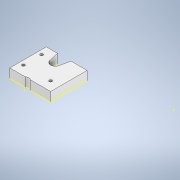
# Autodesk Inventor part: delrin for sides
Saved by Autodesk Inventor 2020.1 (Build 241239000, 239)
## iProperties
Created: 2019-11-10
Part Number: delrin for sides
Material: UHMW, White
Document SubType Name: Modeling
Designer: amirs
Density: 0.94 g/cm^3
Appearance: Smooth - White
Mass: 4.35466 g
Surface Area: 23.8857 cm^2
Volume: 4.63262 cm^3
Author: amirs
Autodesk Inventor part; units mm, degrees
ref_plane "YZ Plane" through (0, 0, 0) normal (1, 0, 0) x (0, 1, 0)
ref_plane "XZ Plane" through (0, 0, 0) normal (0, 1, 0) x (-1, 0, 0)
ref_plane "XY Plane" through (0, 0, 0) normal (0, 0, 1) x (1, 0, 0)
sketch "Sketch1" plane through (0, 0, 0) normal (0, 1, 0) x (-1, 0, 0)
  circle A0 centre (73.1106, 19.0179) radius 0.9652
  circle A1 centre (73.1106, 31.7179) radius 0.9652
  circle A2 centre (54.1114, 31.7179) radius 0.9652
  line L0 (58.8995, 12.6679) -> (60.5161, 19.7267)
  arc A3 (66.7058, 19.7267) -> (60.5161, 19.7267) centre (63.611, 19.0179) ccw
  line L1 (66.7058, 19.7267) -> (68.3224, 12.6679)
  arc A4 (61.706, 38.0679) -> (65.516, 38.0679) centre (63.611, 40.6079) ccw
  line L2 (79.486, 38.0679) -> (79.486, 12.6679) construction
  line L3 (47.736, 12.6679) -> (47.736, 38.0679)
  line L4 (47.736, 38.0679) -> (61.706, 38.0679)
  line L5 (65.516, 38.0679) -> (79.486, 38.0679) construction
  line L6 (79.486, 12.6679) -> (68.3224, 12.6679) construction
  line L7 (58.8995, 12.6679) -> (47.736, 12.6679)
  line L8 (76.184, 38.0679) -> (76.184, 12.6679)
  line L9 (65.516, 38.0679) -> (76.184, 38.0679)
  line L10 (68.3224, 12.6679) -> (76.184, 12.6679)
  point P0 (0, 0)
  dimension "d9" = 1.9304
  dimension "d10" = 25.4
  dimension "d11" = 31.75
  dimension "d14" = 18.9992
  dimension "d15" = 6.3754
  dimension "d16" = 15.875
  dimension "d17" = 15.875
  dimension "d18" = 28.448
  constraints: 22 end point, 5 centre point, 5 parallel, 4 perpendicular, 4 point on circle, 2 equal radius, 2 horizontal, 2 point on line, 1 collinear, 1 vertical alignment
  measures "d9" diameter of A2
  measures "d10" distance of L2.start L2.end
  measures "d11" distance between parallel lines of L2 L3
  measures "d14" distance of A1.centre A2.centre
  measures "d15" distance from line of L3 A2.centre
  measures "d16" distance from line of L3 A4.centre
  measures "d17" distance from line of L3 A3.centre
  measures "d18" distance between parallel lines of L3 L8
extrude "Extrusion1" add sketch "Sketch1" along normal blind 6.35
sketch "Sketch3" plane through (0, 0, 0) normal (0, -1, 0) x (1, 0, 0)
  arc A0 (-60.5161, 19.7267) -> (-66.7058, 19.7267) centre (-63.611, 19.0179) ccw projected
  line L0 (-58.8995, 12.6679) -> (-60.5161, 19.7267) projected
  line L1 (-47.736, 12.6679) -> (-58.8995, 12.6679) projected
  line L2 (-47.736, 38.0679) -> (-47.736, 12.6679) projected
  line L3 (-61.706, 38.0679) -> (-47.736, 38.0679) projected
  arc A1 (-65.516, 38.0679) -> (-61.706, 38.0679) centre (-63.611, 40.6079) ccw projected
  line L4 (-76.184, 38.0679) -> (-65.516, 38.0679) projected
  line L5 (-76.184, 12.6679) -> (-76.184, 38.0679) projected
  line L6 (-68.3224, 12.6679) -> (-76.184, 12.6679) projected
  line L7 (-66.7058, 19.7267) -> (-68.3224, 12.6679) projected
  circle A2 centre (-54.1114, 31.7179) radius 0.9652 projected
  circle A3 centre (-73.1106, 31.7179) radius 0.9652 projected
  circle A4 centre (-73.1106, 19.0179) radius 0.9652 projected
  point P0 (0, 0)
body "Solid1"
